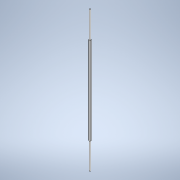
# Autodesk Inventor part: tuboSolido12.7x1240
Saved by Autodesk Inventor 2021 (Build 250183000, 183)
## iProperties
Created: 2026-06-09
Part Number: tuboSolido12.7x1240
Material: Generic
Document SubType Name: Modeling
Designer: nelso
Density: 1 g/cm^3
Appearance: Default
Author: nelso
Autodesk Inventor part; units mm, degrees
ref_plane "YZ Plane" through (0, 0, 0) normal (1, 0, 0) x (0, 1, 0)
ref_plane "XZ Plane" through (0, 0, 0) normal (0, 1, 0) x (-1, 0, 0)
ref_plane "XY Plane" through (0, 0, 0) normal (0, 0, 1) x (1, 0, 0)
sketch "Sketch2" plane through (0, 0, 0) normal (0, 1, 0) x (-1, 0, 0)
  line L0 (8, -4.6188) -> (0, -9.2376)
  line L1 (0, -9.2376) -> (-8, -4.6188)
  line L2 (-8, -4.6188) -> (-8, 4.6188)
  line L3 (-8, 4.6188) -> (0, 9.2376)
  line L4 (0, 9.2376) -> (8, 4.6188)
  line L5 (8, 4.6188) -> (8, -4.6188)
  point P0 (0, 0)
  point P1 (0, 0)
  dimension "d3" = 16
  constraints: 12 end point, 1 coincident, 13 other
  measures "d3" distance between parallel lines of L2 L5
extrude "Extrusion2" add sketch "Sketch2" along normal mid plane 774
sketch "Sketch3" plane through (0, 0, 0) normal (0, 1, 0) x (-1, 0, 0)
  circle A0 centre (0, 0) radius 6
  dimension "d6" = 12
  constraints: 1 centre point, 1 coincident
  measures "d6" diameter of A0
extrude "Extrusion3" add sketch "Sketch3" along normal mid plane 1240
body "Solid2"
